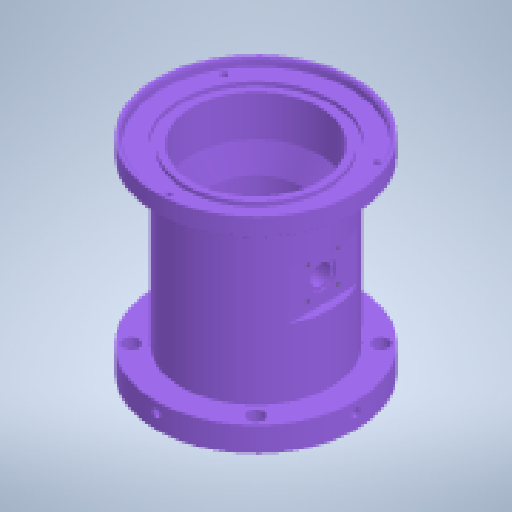
# Autodesk Inventor part: 12
Saved by Autodesk Inventor 2023 (Build 270158000, 158)
## iProperties
Created: 2021-11-02
Part Number: 12
Material: Steel, Galvanized
Document SubType Name: Modeling
Designer: vinicius.miguel
Density: 7.85 g/cm^3
Appearance: Violet
Mass: 1248.53 g
Surface Area: 959.178 cm^2
Volume: 462.417 cm^3
Author: vinicius.miguel
Autodesk Inventor part; units mm, degrees
sketch "Sketch1" plane through (0, 0, 0) normal (0, 0, 1) x (1, 0, 0)
  line L0 (0, 0) -> (0, 14)
  line L1 (18, 12) -> (18, 14)
  line L2 (27.5, 4) -> (35, 4)
  line L3 (60, 0) -> (60, 12)
  line L4 (18, 14) -> (41.45, 14)
  line L5 (41.45, 14) -> (41.45, 12)
  line L6 (41.45, 12) -> (60, 12)
  line L7 (35, 4) -> (35, 0)
  line L8 (41.45, 0) -> (41.45, 2)
  line L9 (41.45, 2) -> (44.45, 2)
  line L10 (44.45, 2) -> (44.45, 0)
  line L11 (35, 0) -> (39, 0)
  line L12 (41.45, -4.213) -> (41.45, -4.213)
  line L13 (39, 0) -> (41.45, 0)
  line L14 (44.45, 0) -> (60, 0)
  line L15 (18, 12) -> (19, 12)
  line L16 (19, 12) -> (19, 13)
  line L17 (19, 13) -> (21, 13)
  line L18 (21, 13) -> (21, 12)
  line L19 (21, 12) -> (27.5, 12)
  line L20 (27.5, 12) -> (27.5, 4)
  line L21 (18, 14) -> (18, 18)
  line L22 (18, 18) -> (27.5, 18)
  line L23 (27.5, 18) -> (31.5, 14)
  line L24 (39, 0) -> (39, -2)
  line L25 (39, -2) -> (41.45, -2)
  line L26 (41.45, -2) -> (41.45, 0)
  dimension "d17" = 36
  dimension "d70" = 38
  dimension "d71" = 2
  dimension "d72" = 1
  dimension "d73" = 8
  dimension "d74" = 3
  dimension "d75" = 2
  dimension "d76" = 55
  dimension "d77" = 70
  dimension "d78" = 4
  dimension "d80" = 120
  dimension "d81" = 82.9
  dimension "d82" = 2
  dimension "d83" = 82.9
  dimension "d84" = 12
  dimension "d94" = 135
  dimension "d95" = 6
  dimension "d112" = 78
  dimension "d113" = 2
  constraints: 54 end point, 16 perpendicular, 5 horizontal alignment, 5 point on line, 5 vertical, 2 horizontal, 1 vertical alignment
  measures "d17" diameter of L1 L0
  measures "d70" diameter of L16 L0
  measures "d71" distance of L16.end L17.end
  measures "d72" distance of L15.end L16.end
  measures "d73" distance of L19.end L2.start
  measures "d74" distance of L8.end L9.end
  measures "d75" distance of L9.end L10.end
  measures "d76" diameter of L20 L0
  measures "d77" diameter of L7 L0
  measures "d78" distance of L2.end L7.end
  measures "d80" diameter of L3 L0
  measures "d81" diameter of L8 L0
  measures "d82" distance of L4.end L5.end
  measures "d83" diameter of L5 L0
  measures "d84" distance of L3.start L3.end
  measures "d94" angle of L23 L22
  measures "d95" distance between parallel lines of L15 L22
  measures "d112" diameter of L24 L0
  measures "d113" distance of L11.end L24.end
revolve "Revolution1" add sketch "Sketch1" angle 360 about axis through (0, 0, 0) along (0, 1, 0)
sketch "Sketch9" plane through (0, 0, 0) normal (0, 0, 1) x (1, 0, 0)
  line L0 (-60, 12) -> (60, 12) projected
  line L1 (-45, 12) -> (-45, 112.8)
  line L2 (-41.45, 14) -> (-41.45, 12) projected
  line L3 (-31.5, 14) -> (31.5, 14) projected
  line L4 (-41.45, 14) -> (41.45, 14) projected
  line L5 (-27.5, 18) -> (27.5, 18) projected
  line L6 (-31.5, 14) -> (31.5, 14) projected
  line L7 (-27.5, 18) -> (-31.5, 14) projected
  line L8 (-18, 18) -> (18, 18) projected
  line L9 (-18, 12) -> (-18, 18) projected
  line L10 (-27.5, 18) -> (-27.5, 83)
  line L11 (-27.5, 83) -> (-38.5, 94)
  line L12 (-38.5, 94) -> (-38.5, 118.8)
  line L13 (-39, -2) -> (39, -2) projected
  line L14 (0, -2) -> (0, 99.1693) construction
  line L15 (-38.5, 118.8) -> (-42.5, 118.8)
  line L16 (-42.5, 118.8) -> (-42.5, 116.3)
  line L17 (-42.5, 116.3) -> (-46, 116.3)
  line L18 (-46, 116.3) -> (-46, 118.8)
  line L19 (-46, 118.8) -> (-57, 118.8)
  line L20 (-57, 118.8) -> (-57, 122.3)
  line L21 (-57, 122.3) -> (-58, 123.3)
  line L22 (-58, 123.3) -> (-60, 123.3)
  line L23 (-60, 123.3) -> (-60, 112.8)
  line L24 (-60, 112.8) -> (-45, 112.8)
  line L25 (-27.5, 18) -> (27.5, 18) projected
  line L26 (-27.5, 27.5) -> (-18, 18)
  line L27 (-18, 18) -> (-18, 18)
  line L28 (-18, 12) -> (-18, 18) projected
  point P0 (0, 0)
  dimension "d114" = 90
  dimension "d115" = 135
  dimension "d117" = 100.8
  dimension "d118" = 10.5
  dimension "d119" = 2
  dimension "d120" = 120
  dimension "d121" = 77
  dimension "d122" = 114
  dimension "d123" = 135
  dimension "d124" = 6
  dimension "d125" = 3.5
  dimension "d126" = 2.5
  dimension "d127" = 85
  dimension "d132" = 65
  dimension "d164" = 135
  dimension "d165" = 0
  constraints: 34 end point, 6 perpendicular, 5 point on line, 3 parallel, 3 vertical, 1 coincident, 1 collinear, 1 horizontal, 1 midpoint
  measures "d114" diameter of L1 L14
  measures "d115" angle of L10 L11
  measures "d117" distance from line of L24 L1.start
  measures "d118" distance of L22.end L23.end
  measures "d119" distance of L21.end L22.end
  measures "d120" diameter of L23 L14
  measures "d121" diameter of L12 L14
  measures "d122" diameter of L20 L14
  measures "d123" angle of L20 L21
  measures "d124" distance between parallel lines of L24 L19
  measures "d125" distance of L16.end L17.end
  measures "d126" distance of L17.end L18.end
  measures "d127" diameter of L16 L14
  measures "d132" distance of L10.start L10.end
  measures "d164" angle of L27 L26
  measures "d165" distance of L26.end L9.end
revolve "Revolution2" add sketch "Sketch9" angle 360 about axis through (0, -2, 0) along (0, 1, 0) contours L1 L24 L23 L22 L21 L20 L19 L18 L17 L16 L15 L12 L11 L10 L7 L4 L2 L0 | L5 L10 L26
ref_plane "Work Plane1" through (60, 6, 0) normal (1, 0, 0) x (0, 1, 0)
sketch "Sketch2" plane through (60, 6, 0) normal (1, 0, 0) x (0, 1, 0)
  line L0 (6, 60) -> (6, -60) projected
  line L1 (6, 27.5) -> (6, -27.5) projected
  line L2 (-2, 27.5) -> (-2, -27.5) projected
  line L3 (6, 21) -> (6, -21) projected
  point P0 (-6, 0)
  point P1 (3, 0)
  point P2 (6, 0)
  point P3 (3, 0)
  dimension "d129" = 3
  constraints: 1 coincident, 1 horizontal alignment, 1 midpoint
  measures "d129" distance of point (3, 0) point (6, 0)
hole "Hole1" at (60, 9, 0) direction (-1, 0, 0) diameter 3.242 depth 40 tip angle 118 counterbore diameter 5 counterbore depth 20 thread size "M4x0.7" class "6H" standard "ANSI Metric M Profile"
pattern_circular "Circular Pattern1" count 4 over 360 about axis through (0, 6, 0) along (0, -1, 0) of "Hole1"
sketch "Sketch7" plane through (0, 12, 0) normal (0, -1, 0) x (1, 0, 0)
  point P0 (0, 0)
  point P1 (23, 0)
  dimension "d86" = 23
  constraints: 1 horizontal alignment
  measures "d86" distance of point (23, 0) point (0, 0)
hole "Hole4" at (23, 12, 0) direction (0, 1, 0) diameter 1.567 depth 6 tip angle 118 thread size "M2x0.4" class "6H" standard "ISO Metric profile"
pattern_circular "Circular Pattern3" count 4 over 360 about axis through (0, 6, 0) along (0, -1, 0) of "Hole4"
sketch "Sketch8" plane through (0, 12, 0) normal (0, 1, 0) x (1, 0, 0)
  line L0 (0, 0) -> (54.0517, 0)
  point P0 (37.4767, 37.4767)
  dimension "d99" = 53
  dimension "d100" = 45
  constraints: 2 end point, 1 horizontal
  measures "d99" distance of point (37.477, 37.477) L0.start
hole "Hole5" at (37.4767, 12, -37.4767) direction (0, -1, 0) diameter 10 end through all
pattern_circular "Circular Pattern4" count 4 over 360 about axis through (0, 6, 0) along (0, -1, 0) of "Hole5"
sketch "Sketch10" plane through (0, 12, 0) normal (0, 1, 0) x (1, 0, 0)
  circle A0 centre (-37.4767, 37.4767) radius 5 projected
  circle A1 centre (-37.4767, -37.4767) radius 5 projected
  circle A2 centre (37.4767, -37.4767) radius 5 projected
  circle A3 centre (37.4767, 37.4767) radius 5 projected
  circle A4 centre (0, 0) radius 45 projected
  circle A5 centre (0, 0) radius 60 projected
extrude "Extrusion2" add sketch "Sketch10" along normal blind 3 contours A0 | A1 | A2 | A3 | A5
ref_plane "Work Plane4" through (0, 62.4, -45) normal (0, 0, 1) x (1, 0, 0)
sketch "Sketch13" plane through (0, 62.4, -45) normal (0, 0, 1) x (1, 0, 0)
  line L0 (27.5, 20.6) -> (-27.5, 20.6) construction
  line L1 (0, 20.6) -> (0, -47.4) construction
  line L2 (60, -47.4) -> (-60, -47.4) projected
  circle A0 centre (0, -14.9) radius 32.5
  line L3 (64.369, -47.4) -> (-64.369, -47.4)
  line L4 (-64.369, -47.4) -> (-64.369, 17.6)
  line L5 (-64.369, 17.6) -> (64.369, 17.6)
  line L6 (64.369, 17.6) -> (64.369, -47.4)
  line L7 (64.369, -47.4) -> (-64.369, 17.6) construction
  line L8 (-64.369, -47.4) -> (64.369, 17.6) construction
  point P0 (0, -62.4)
  point P1 (59.4175, -47.4)
  point P2 (0, 17.6)
  point P3 (0, -47.4)
  point P4 (-59.4175, -47.4)
  dimension "d142" = 65
  constraints: 14 end point, 4 midpoint, 2 parallel, 2 tangent, 1 centre point, 1 horizontal, 1 perpendicular, 1 point on line, 1 vertical
  measures "d142" diameter of A0
extrude "Extrusion4" cut sketch "Sketch13" along normal blind 12
sketch "Sketch14" plane through (0, 62.4, -33) normal (0, 0, -1) x (-1, 0, 0)
  line L0 (-30.5941, -47.4) -> (-30.5941, 17.6) projected
  line L1 (30.5941, -47.4) -> (-30.5941, -47.4) projected
  line L2 (30.5941, 17.6) -> (30.5941, -47.4) projected
  line L3 (-30.5941, 17.6) -> (30.5941, 17.6) projected
  circle A0 centre (0, -14.9) radius 20
  line L4 (30.5941, 17.6) -> (-30.5941, 17.6) projected
  point P0 (0, -62.4)
  point P1 (-30.5941, -14.9)
  point P2 (0, 17.6)
  dimension "d143" = 40
  constraints: 2 midpoint, 1 centre point, 1 horizontal alignment, 1 vertical alignment
  measures "d143" diameter of A0
extrude "Extrusion5" cut sketch "Sketch14" against normal blind 20 contours A0
sketch "Sketch3" plane through (0, 0, 0) normal (0, -1, 0) x (1, 0, 0)
  line L0 (0, 0) -> (-65.7785, -23.9414) construction
  line L1 (-4.7883, 13.1557) -> (-70.5668, -10.7857)
  line L2 (-60.9902, -37.0971) -> (4.7883, -13.1557)
  arc A0 (4.7883, -13.1557) -> (-4.7883, 13.1557) centre (0, 0) ccw
  arc A1 (-70.5668, -10.7857) -> (-60.9902, -37.0971) centre (-65.7785, -23.9414) ccw
  line L3 (0, 0) -> (70, 0) construction
  point P0 (-32.8892, -11.9707)
  dimension "d40" = 70
  dimension "d42" = 28
  dimension "d111" = 160
  constraints: 10 end point, 4 point on circle, 4 tangent, 2 centre point, 1 equal length, 1 horizontal, 1 midpoint, 1 parallel
  measures "d40" distance of L0.start L0.end
  measures "d42" diameter of A1
  measures "d111" angle of L3 L0
extrude "Extrusion1" cut sketch "Sketch3" along normal blind 4 and the other way blind 4
sketch "Sketch16" plane through (0, 62.4, -33) normal (0, 0, -1) x (-1, 0, 0)
  circle A0 centre (0, -14.9) radius 20 projected
  circle A1 centre (0, -14.9) radius 22
  point P0 (0, -62.4)
  point P1 (-1.4844, 2.5448)
  point P2 (-1.4844, -37.3448)
  dimension "d150" = 2
  constraints: 1 centre point, 1 other
extrude "Extrusion6" cut sketch "Sketch16" against normal blind 1 contours A0 | A1
sketch "Sketch17" plane through (0, 62.4, -33) normal (0, 0, -1) x (-1, 0, 0)
  circle A0 centre (0, -14.9) radius 20 projected
  line L0 (-19.0919, 4.1919) -> (19.0919, 4.1919)
  line L1 (19.0919, 4.1919) -> (19.0919, -33.9919)
  line L2 (19.0919, -33.9919) -> (-19.0919, -33.9919)
  line L3 (-19.0919, -33.9919) -> (-19.0919, 4.1919)
  line L4 (-19.0919, 4.1919) -> (19.0919, -33.9919) construction
  line L5 (19.0919, 4.1919) -> (-19.0919, -33.9919) construction
  circle A1 centre (0, -14.9) radius 29.75
  point P0 (0, -62.4)
  point P1 (-1.8987, 2.5097)
  point P2 (-1.8987, -37.3097)
  dimension "d154" = 59.5
  dimension "d156" = 54
  constraints: 12 end point, 5 coincident, 2 midpoint, 2 parallel, 2 perpendicular, 1 centre point, 1 horizontal, 1 other
  measures "d154" diameter of A1
  measures "d156" distance of L0.start L1.end
hole "Hole6" at (19.0919, 66.5919, -33) at (-19.0919, 66.5919, -33) at (-19.0919, 28.4081, -33) at (19.0919, 28.4081, -33) direction (0, 0, 1) diameter 2.459 depth 8.8 tip angle 118 thread size "M3x0.5" class "6H" standard "ISO Metric profile"
ref_plane "Work Plane5" through (45, 62.4, 0) normal (1, 0, 0) x (0, 1, 0)
sketch "Sketch18" plane through (45, 62.4, 0) normal (1, 0, 0) x (0, 1, 0)
  spline S0 degree 3 poles (8.1, 6) (8.8603, 6) (9.6666, 5.8468) (11.1427, 5.2327) (11.8132, 4.772) (12.8718, 3.7135) (13.3326, 3.0429) (13.9469, 1.5663) (14.1, 0.7599) (14.1, -0.7599) (13.9469, -1.5663) (13.3326, -3.0429) (12.8718, -3.7135) (11.8132, -4.772) (11.1427, -5.2327) (9.6666, -5.8468) (8.8603, -6) (7.3397, -6) (6.5334, -5.8468) (5.0573, -5.2327) (4.3868, -4.772) (3.3282, -3.7135) (2.8674, -3.0429) (2.2531, -1.5663) (2.1, -0.7599) (2.1, 0.7599) (2.2531, 1.5663) (2.8674, 3.0429) (3.3282, 3.7135) (4.3868, 4.772) (5.0573, 5.2327) (6.5334, 5.8468) (7.3397, 6) (8.1, 6) knots 0 0 0 0 0.228087 0.228087 0.456173 0.456173 0.68414 0.68414 0.912108 0.912108 1.140075 1.140075 1.368043 1.368043 1.596129 1.596129 1.824216 1.824216 2.052302 2.052302 2.280389 2.280389 2.508356 2.508356 2.736323 2.736323 2.964291 2.964291 3.192258 3.192258 3.420345 3.420345 3.648431 3.648431 3.648431 3.648431 projected
  line L0 (23.1, 57.3709) -> (-6.9, 57.3709)
  line L1 (-6.9, 57.3709) -> (-6.9, -57.3709)
  line L2 (-6.9, -57.3709) -> (23.1, -57.3709)
  line L3 (23.1, -57.3709) -> (23.1, 57.3709)
  line L4 (23.1, 57.3709) -> (-6.9, -57.3709) construction
  line L5 (-6.9, 57.3709) -> (23.1, -57.3709) construction
  point P0 (-62.4, 0)
  point P1 (8.1, 6)
  point P2 (8.1, 0)
  point P3 (8.1, 0)
  point P4 (8.1, 0)
  dimension "d166" = 30
  constraints: 12 end point, 4 midpoint, 2 parallel, 1 horizontal, 1 horizontal alignment, 1 perpendicular, 1 vertical alignment
  measures "d166" distance of L2.end L1.end
extrude "Extrusion7" cut sketch "Sketch18" against normal blind 5 contours S0 | L3 L2 L1 L0
sketch "Sketch19" plane through (40, 62.4, 0) normal (1, 0, 0) x (0, 0, -1)
  line L0 (-20.6155, -6.9) -> (-20.6155, 23.1) projected
  line L1 (20.6155, -6.9) -> (-20.6155, -6.9) projected
  line L2 (20.6155, 23.1) -> (20.6155, -6.9) projected
  line L3 (-20.6155, 23.1) -> (20.6155, 23.1) projected
  circle A0 centre (0, 8.1) radius 6
  line L4 (20.6155, 23.1) -> (-20.6155, 23.1) projected
  point P0 (0, -62.4)
  point P1 (0, 23.1)
  point P2 (20.6155, 8.1)
  dimension "d169" = 12
  constraints: 2 midpoint, 1 centre point, 1 horizontal alignment, 1 vertical alignment
  measures "d169" diameter of A0
extrude "Extrusion8" cut sketch "Sketch19" against normal blind 15 contours A0
sketch "Sketch20" plane through (40, 62.4, 0) normal (1, 0, 0) x (0, 0, -1)
  circle A0 centre (0, 8.1) radius 6 projected
  circle A1 centre (0, 8.1) radius 8
  point P0 (0, -62.4)
  dimension "d172" = 2
  constraints: 1 centre point
  measures "d172" radial gap between concentric circles of A0 A1
extrude "Extrusion9" cut sketch "Sketch20" against normal blind 1
sketch "Sketch21" plane through (40, 62.4, 0) normal (1, 0, 0) x (0, 0, -1)
  circle A0 centre (0, 8.1) radius 6 projected
  line L0 (-8.8709, 17.603) -> (8.8709, 17.603)
  line L1 (8.8709, 17.603) -> (8.8709, -1.403)
  line L2 (8.8709, -1.403) -> (-8.8709, -1.403)
  line L3 (-8.8709, -1.403) -> (-8.8709, 17.603)
  line L4 (-8.8709, 17.603) -> (8.8709, -1.403) construction
  line L5 (8.8709, 17.603) -> (-8.8709, -1.403) construction
  circle A1 centre (0, 8.1) radius 14.75
  point P0 (0, -62.4)
  dimension "d175" = 29.5
  dimension "d176" = 26
  constraints: 12 end point, 5 coincident, 2 midpoint, 2 parallel, 1 centre point, 1 horizontal, 1 perpendicular
  measures "d175" diameter of A1
  measures "d176" distance of L0.start L1.end
hole "Hole7" at (40, 80.003, 8.8709) at (40, 80.003, -8.8709) at (40, 60.997, -8.8709) at (40, 60.997, 8.8709) direction (-1, 0, 0) diameter 2.459 depth 8.8 tip angle 118 thread size "M3x0.5" class "6H" standard "ISO Metric profile"
chamfer "Chamfer1" distance 5 angle 45 1 edges at (45, 112.8, 0)
sketch "Sketch22" plane through (0, 118.8, 0) normal (0, 1, 0) x (1, 0, 0)
  circle A0 centre (0, 0) radius 46 projected
  circle A1 centre (0, 0) radius 57 projected
  point P0 (0, -53)
  dimension "d187" = 53
  constraints: 1 vertical alignment
  measures "d187" distance of point (0, 0) point (0, -53)
hole "Hole8" at (0, 118.8, 53) direction (0, -1, 0) diameter 3.6 depth 8.8 tip angle 118 clearance for "Countersunk Flat Head Screw DIN EN ISO 2009" size "M3" standard "DIN"
pattern_circular "Circular Pattern5" count 3 over 360 about axis through (0, 62.4, 0) along (0, 1, 0) of "Hole8"
sketch "Sketch23" plane through (0, 15, 0) normal (0, 1, 0) x (1, 0, 0)
  line L0 (37.4767, -37.4767) -> (-37.4767, -37.4767)
  line L1 (-37.4767, -37.4767) -> (-37.4767, 37.4767)
  line L2 (-37.4767, 37.4767) -> (37.4767, 37.4767)
  line L3 (37.4767, 37.4767) -> (37.4767, -37.4767)
  line L4 (37.4767, -37.4767) -> (-37.4767, 37.4767) construction
  line L5 (-37.4767, -37.4767) -> (37.4767, 37.4767) construction
  point P0 (0, 0)
  dimension "d200" = 106
  constraints: 12 end point, 2 midpoint, 2 parallel, 2 perpendicular, 1 coincident, 1 horizontal
  measures "d200" distance of L0.start L1.end
hole "Hole9" at (-37.4767, 15, -37.4767) direction (0, -1, 0) diameter 9 end through all clearance for "Countersunk Flat Head Screw DIN EN ISO 2009" size "M8" standard "DIN"
pattern_circular "Circular Pattern6" count 4 over 360 about axis through (0, 62.4, 0) along (0, 1, 0) of "Hole9"
chamfer "Chamfer2" distance 0.25 angle 45 5 edges at (60, 123.3, 0) (60, 112.8, 0) (-60, 15, 0) (-3.405, 0, 59.9033) (17.2885, 0, -57.4553)
equation "\"d83\" = d81"
body "Solid1"
